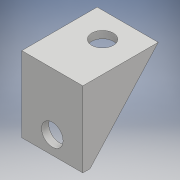
# Autodesk Inventor part: Triangulo
Saved by Autodesk Inventor 2018.3 (Build 223284000, 284)
## iProperties
Created: 2021-02-08
Part Number: Triangulo
Material: Genérico
Document SubType Name: Modeling
Designer: SERGIO ROMO
Density: 1 g/cm^3
Appearance: Valor por defecto
Author: SERGIO ROMO
Autodesk Inventor part; units mm, degrees
ref_plane "YZ Plane" through (0, 0, 0) normal (1, 0, 0) x (0, 1, 0)
ref_plane "XZ Plane" through (0, 0, 0) normal (0, 1, 0) x (-1, 0, 0)
ref_plane "XY Plane" through (0, 0, 0) normal (0, 0, 1) x (1, 0, 0)
sketch "Boceto2" plane through (0, 0, 0) normal (0, 1, 0) x (-1, 0, 0)
  line L0 (0, 0) -> (-17, 0)
  line L1 (-17, 0) -> (-17, -21)
  line L2 (-17, -21) -> (0, -21)
  line L3 (0, -21) -> (0, 0)
  dimension "d0" = 17
  dimension "d1" = 21
  dimension "d2" = 17
  constraints: 8 end point, 2 perpendicular, 1 horizontal
  measures "d0" distance of L0.start L0.end
  measures "d1" distance of L0.end L1.end
  measures "d2" distance of L1.end L2.end
extrude "Extrusión1" add sketch "Boceto2" along normal blind 2
sketch "Boceto3" plane through (0, 2, 0) normal (0, 1, 0) x (1, 0, 0)
  line L0 (0, 0) -> (17, 0) projected
  line L1 (0, 0) -> (0, 21)
  line L2 (0, 21) -> (0, 0) projected
  line L3 (0, 21) -> (17, 21)
  line L4 (17, 0) -> (17, 21) projected
  line L5 (0, 0) -> (17, 0)
  line L6 (17, 0) -> (17, 21)
  dimension "d5" = 21
  constraints: 8 end point, 2 perpendicular, 2 point on line, 1 horizontal
  measures "d5" distance of L0.start L1.end
extrude "Extrusión3" add sketch "Boceto3" along normal blind 19
sketch "Boceto5" plane through (0, 21, 0) normal (0, 1, 0) x (1, 0, 0)
  line L0 (17, 21) -> (0, 21) projected
  line L1 (2, 21) -> (2, 2)
  line L2 (2, 2) -> (15, 2)
  line L3 (15, 2) -> (15, 21)
  line L4 (15, 21) -> (2, 21)
  point P0 (0, 0)
  constraints: 8 end point, 3 perpendicular, 1 point on line
extrude "Extrusión5" cut sketch "Boceto5" against normal blind 19
sketch "Boceto6" plane through (17, 0, 0) normal (1, 0, 0) x (0, 0, -1)
  line L0 (0, 0) -> (21, 0) projected
  line L1 (0, 21) -> (21, 21) projected
  line L2 (21, 2) -> (0, 21)
  line L3 (0, 21) -> (21, 21)
  line L4 (21, 21) -> (21, 2)
  constraints: 6 end point, 1 collinear, 1 perpendicular
extrude "Extrusión6" cut sketch "Boceto6" against normal blind 19
sketch "Boceto7" plane through (0, 2, 0) normal (0, 1, 0) x (1, 0, 0)
  line L0 (0, 0) -> (17, 0) projected
  circle A0 centre (8.5, 16) radius 3
  constraints: 1 centre point
extrude "Extrusión7" cut sketch "Boceto7" against normal blind 19
sketch "Boceto8" plane through (15, 2, -2) normal (0, 0, -1) x (-1, 0, 0)
  line L0 (-2, -2) -> (15, -2) projected
  circle A0 centre (6.5, 12) radius 3
  constraints: 1 centre point
extrude "Extrusión8" cut sketch "Boceto8" against normal blind 19
